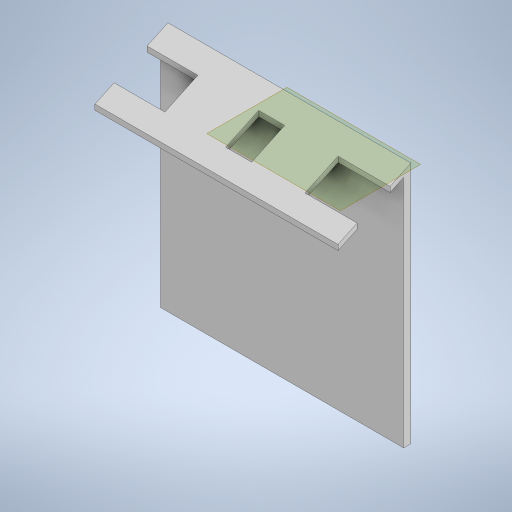
# Autodesk Inventor part: Test rampy
Saved by Autodesk Inventor 2024 (Build 280153000, 153)
## iProperties
Created: 2023-09-07
Part Number: Test rampy
Material: Všeobecné
Document SubType Name: Modeling
Designer: jaryj
Density: 1 g/cm^3
Appearance: Výchozí
Author: jaryj
Autodesk Inventor part; units mm, degrees
ref_plane "YZ Plane" through (0, 0, 0) normal (1, 0, 0) x (0, 1, 0)
ref_plane "XZ Plane" through (0, 0, 0) normal (0, 1, 0) x (-1, 0, 0)
ref_plane "XY Plane" through (0, 0, 0) normal (0, 0, 1) x (1, 0, 0)
sketch "Náčrt1" plane through (0, 0, 0) normal (0, 0, 1) x (1, 0, 0)
  line L0 (0, -50) -> (50, -50)
  line L1 (50, -50) -> (50, 50)
  line L2 (50, 50) -> (0, 50)
  line L3 (0, 50) -> (0, -50)
  point P0 (0, 0)
  point P1 (50, 0)
  point P2 (0, 0)
  dimension "d0" = 50
  dimension "d1" = 100
  constraints: 8 end point, 2 midpoint, 2 parallel, 1 coincident, 1 horizontal, 1 horizontal alignment, 1 perpendicular
  measures "d0" distance of L0.start L0.end
  measures "d1" distance of L0.end L1.end
extrude "Vysunutí1" add sketch "Náčrt1" along normal blind 3
sketch "Náčrt2" plane through (50, -50, 0) normal (1, 0, 0) x (0, 0, -1)
  line L0 (0, 0) -> (0, 100) projected
  line L1 (0, 100) -> (-30, 86.0108)
  line L2 (-30, 86.0108) -> (-30, 83.804)
  line L3 (-30, 83.804) -> (0, 97.7932)
  line L4 (-3, 0) -> (-3, 100) projected
  line L5 (0, 100) -> (-3, 100) projected
  point P0 (0, 50)
  point P1 (-3, 98.6011)
  dimension "d4" = 65
  dimension "d6" = 2
  dimension "d7" = 30
  constraints: 6 end point, 1 point on line, 1 vertical
  measures "d4" angle of L0 L1
  measures "d6" distance between parallel lines of L1 L3
  measures "d7" distance between parallel lines of L0 L2
extrude "Vysunutí2" add sketch "Náčrt2" against normal up to surface (50 mm away) contours L3 L4 L1 L0 | L3 L2 L1 L4
extrude "Vysunutí3" cut sketch "Náčrt2" against normal through all contours L1 L4 L5
ref_plane "Pracovní rovina1" through (50, 50, 0) normal (0, -1, 0) x (1, 0, 0)
mirror "Zrcadlit1" about plane through (0, 0, 0) normal (1, 0, 0)
sketch "Náčrt3" plane through (50, 50, 0) normal (0, -1, 0) x (1, 0, 0)
  line L0 (-12.748, 22.13) -> (-21.41, 22.13)
  line L1 (-21.41, 22.13) -> (-21.41, 8.58)
  line L2 (-21.41, 8.58) -> (-12.748, 8.58)
  line L3 (-12.748, 8.58) -> (-12.748, 22.13)
  line L4 (-54.03, 8.58) -> (-43.38, 8.58)
  line L5 (-43.38, 8.58) -> (-43.38, 22.13)
  line L6 (-43.38, 22.13) -> (-54.03, 22.13)
  line L7 (-54.03, 22.13) -> (-54.03, 8.58)
  line L8 (0, 0) -> (0, 30) projected
  line L9 (0, 0) -> (-50, 0) projected
  line L10 (-79.1, 22.13) -> (-87.762, 22.13)
  line L11 (-87.762, 22.13) -> (-87.762, 8.58)
  line L12 (-87.762, 8.58) -> (-79.1, 8.58)
  line L13 (-79.1, 8.58) -> (-79.1, 22.13)
  line L14 (-100, 0) -> (-100, 30) projected
  line L15 (-87.762, 22.13) -> (-100, 22.13)
  line L16 (-87.762, 8.58) -> (-100, 8.58)
  line L17 (-12.748, 22.13) -> (0, 22.13)
  line L18 (-12.748, 8.58) -> (0, 8.58)
  dimension "d13" = 22.13
  dimension "d14" = 21.97
  dimension "d15" = 8.662
  dimension "d18" = 25.07
  dimension "d19" = 12.238
  dimension "d20" = 10.65
  dimension "d21" = 8.662
  dimension "d22" = 8.58
  constraints: 32 end point, 6 parallel, 6 point on line, 5 perpendicular, 4 horizontal alignment, 3 horizontal
  measures "d13" distance between parallel lines of L6 L9
  measures "d14" distance between parallel lines of L5 L1
  measures "d15" distance between parallel lines of L1 L3
  measures "d18" distance between parallel lines of L13 L7
  measures "d19" distance between parallel lines of L14 L11
  measures "d20" distance between parallel lines of L7 L5
  measures "d21" distance between parallel lines of L11 L13
  measures "d22" distance between parallel lines of L9 L4
extrude "Vysunutí4" cut sketch "Náčrt3" along normal through all
